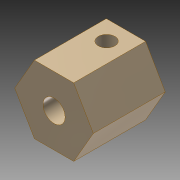
# Autodesk Inventor part: Hub_Hex_12mm
Saved by Autodesk Inventor 2014 SP1 (Build 180222100, 222)
## iProperties
Created: 2015-04-18
Part Number: Hub_Hex_12mm
Material: Polyethylene, Low Density
Document SubType Name: Modeling
Designer: david
Density: 0.894 g/cm^3
Appearance: Smooth - Off-White
Mass: 1.307 g
Surface Area: 10.015 cm^2
Volume: 1.46197 cm^3
Author: david
Autodesk Inventor part; units mm, degrees
ref_plane "YZ Plane" through (0, 0, 0) normal (1, 0, 0) x (0, 1, 0)
ref_plane "XZ Plane" through (0, 0, 0) normal (0, 1, 0) x (-1, 0, 0)
ref_plane "XY Plane" through (0, 0, 0) normal (0, 0, 1) x (1, 0, 0)
sketch "Sketch1" plane through (0, 0, 0) normal (0, 1, 0) x (-1, 0, 0)
  line L0 (7.1014, 0) -> (3.5507, -6.15)
  line L1 (3.5507, -6.15) -> (-3.5507, -6.15)
  line L2 (-3.5507, -6.15) -> (-7.1014, 0)
  line L3 (-7.1014, 0) -> (-3.5507, 6.15)
  line L4 (-3.5507, 6.15) -> (3.5507, 6.15)
  line L5 (3.5507, 6.15) -> (7.1014, 0)
  line L6 (0, 0) -> (25.8005, 0) construction
  dimension "d0" = 12.3
  constraints: 14 end point, 1 coincident, 1 horizontal, 1 point on line, 13 other
  measures "d0" distance between parallel lines of L1 L4
extrude "Extrusion1" add sketch "Sketch1" along normal blind 13
sketch "Sketch2" plane through (0, 13, 0) normal (0, 1, 0) x (1, 0, 0)
  line L0 (3.5507, 6.15) -> (-3.5507, 6.15) projected
  line L1 (-1.8974, 1.3) -> (1.8974, 1.3)
  line L2 (-1.8974, -1.3) -> (1.8974, -1.3)
  arc A0 (-1.8974, 1.3) -> (-1.8974, -1.3) centre (0, 0) ccw
  arc A1 (1.8974, -1.3) -> (1.8974, 1.3) centre (0, 0) ccw
  dimension "d4" = 2.6
  dimension "d5" = 2.3
  dimension "d6" = 2.3
  constraints: 4 end point, 4 point on circle, 3 parallel, 2 centre point, 1 coincident
  measures "d4" distance between parallel lines of L2 L1
  measures "d5" radius of A0
  measures "d6" radius of A1
extrude "Extrusion2" cut sketch "Sketch2" against normal blind 9
sketch "Sketch6" plane through (0, 0, 0) normal (0, -1, 0) x (1, 0, 0)
  circle A0 centre (0, 0) radius 2
  dimension "d16" = 4
  constraints: 1 centre point, 1 coincident
  measures "d16" diameter of A0
extrude "Extrusion5" cut sketch "Sketch6" against normal up to surface (4 mm away)
sketch "Sketch7" plane through (3.5507, 0, -6.15) normal (0, 0, -1) x (-1, 0, 0)
  line L0 (0, 13) -> (7.1014, 13) projected
  line L1 (0, 0) -> (0, 13) projected
  circle A0 centre (3.5507, 9.5) radius 1.5
  line L2 (3.5507, 0) -> (3.5507, 15.2107) construction
  dimension "d19" = 3
  dimension "d20" = 3.5
  constraints: 2 end point, 1 centre point, 1 parallel, 1 point on line
  measures "d19" diameter of A0
  measures "d20" distance from line of L0 A0.centre
extrude "Extrusion6" cut sketch "Sketch7" against normal through all
equation "\"Plastic_Reduction_Margin\" = 0.3"
body "Solid1"
